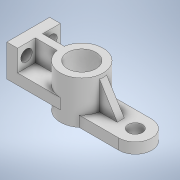
# Autodesk Inventor part: Exercise03
Saved by Autodesk Inventor 2021 (Build 250183000, 183)
## iProperties
Created: 2022-03-19
Part Number: Exercise03
Material: Generic
Document SubType Name: Modeling
Designer: User
Density: 1 g/cm^3
Appearance: Default
Author: User
Autodesk Inventor part; units mm, degrees
ref_plane "YZ Plane" through (0, 0, 0) normal (1, 0, 0) x (0, 1, 0)
ref_plane "XZ Plane" through (0, 0, 0) normal (0, 1, 0) x (-1, 0, 0)
ref_plane "XY Plane" through (0, 0, 0) normal (0, 0, 1) x (1, 0, 0)
sketch "Sketch1" plane through (0, 0, 0) normal (0, 1, 0) x (-1, 0, 0)
  circle A0 centre (0, 0) radius 30
  circle A1 centre (0, 0) radius 20
  dimension "d0" = 60
  dimension "d1" = 40
  constraints: 2 centre point, 2 coincident
  measures "d0" diameter of A0
  measures "d1" diameter of A1
extrude "Extrusion1" add sketch "Sketch1" along normal blind 60
sketch "Sketch2" plane through (0, 0, 0) normal (0, -1, 0) x (1, 0, 0)
  circle A0 centre (75, 0) radius 10
  arc A1 (75, -23) -> (75, 23) centre (75, 0) ccw
  circle A2 centre (0, 0) radius 30 projected
  line L0 (19.2614, 23) -> (75, 23)
  line L1 (19.2614, -23) -> (75, -23)
  dimension "d4" = 20
  dimension "d5" = 46
  dimension "d8" = 75
  constraints: 4 end point, 4 point on circle, 2 centre point, 2 parallel, 1 coincident, 1 horizontal, 1 horizontal alignment, 1 tangent
  measures "d4" diameter of A0
  measures "d5" diameter of A1
  measures "d8" distance of A1.centre A2.centre
extrude "Extrusion2" add sketch "Sketch2" against normal blind 15 contours L1 A2 L0 A1
sketch "Sketch3" plane through (0, 15, 0) normal (0, 1, 0) x (1, 0, 0)
  line L0 (-75, -30) -> (0, -30)
  line L1 (0, -30) -> (0, 30)
  line L2 (0, 30) -> (-75, 30)
  line L3 (-75, 30) -> (-75, -30)
  arc A0 (19.2614, 23) -> (19.2614, -23) centre (0, 0) ccw projected
  dimension "d11" = 60
  dimension "d12" = 75
  constraints: 8 end point, 2 parallel, 2 point on circle, 1 horizontal, 1 perpendicular
  measures "d11" distance of L2.end L0.start
  measures "d12" distance of L0.start L0.end
extrude "Extrusion3" add sketch "Sketch3" along normal blind 15 contours L3 L2 A0 L0
sketch "Sketch4" plane through (0, 30, 0) normal (0, 1, 0) x (1, 0, 0)
  line L0 (-75, 30) -> (-60, 30)
  line L1 (-60, 30) -> (-60, -30)
  line L2 (-60, -30) -> (-75, -30)
  line L3 (-75, -30) -> (-75, 30)
  line L4 (0, 30) -> (-75, 30) projected
  line L5 (-75, 30) -> (-75, -30) projected
  line L6 (-75, -30) -> (0, -30) projected
  line L7 (-60, 5) -> (-29.5804, 5)
  line L8 (-29.5804, 5) -> (-29.5804, -5)
  line L9 (-29.5804, -5) -> (-60, -5)
  line L10 (-60, -5) -> (-60, 5)
  circle A0 centre (0, 0) radius 30 projected
  dimension "d15" = 15
  dimension "d16" = 10
  constraints: 16 end point, 4 parallel, 3 collinear, 2 horizontal, 2 perpendicular, 2 point on circle, 1 point on line
  measures "d15" distance between parallel lines of L3 L1
  measures "d16" distance between parallel lines of L7 L9
extrude "Extrusion4" add sketch "Sketch4" along normal blind 30 contours L0 L1 L2 L3 | L7 A0 L9 L1 | L8 A0 picked at (-29.7047, 0.5579)
sketch "Sketch5" plane through (-75, 15, -30) normal (-1, 0, 0) x (0, 0, 1)
  circle A0 centre (12.5, 30) radius 8
  circle A1 centre (47.5, 30) radius 8
  line L0 (60, 0) -> (60, 45) projected
  line L1 (0, 45) -> (60, 45) projected
  point P0 (30, -15)
  dimension "d19" = 16
  dimension "d20" = 35
  dimension "d21" = 12.5
  dimension "d22" = 15
  constraints: 2 centre point, 1 equal radius, 1 horizontal alignment
  measures "d19" diameter of A0
  measures "d20" distance of A1.centre A0.centre
  measures "d21" distance from line of L0 A1.centre
  measures "d22" distance from line of L1 A0.centre
extrude "Extrusion5" cut sketch "Sketch5" against normal up to surface (15 mm away)
sketch "Sketch6" plane through (0, 0, 0) normal (0, 0, 1) x (1, 0, 0)
  line L0 (29.615, 55) -> (29.615, 15)
  line L1 (29.615, 15) -> (54.615, 15)
  line L2 (54.615, 15) -> (29.615, 55)
  line L3 (19.2614, 15) -> (75, 15) projected
  line L4 (29.998, 59.9996) -> (29.998, 15) construction
  point P0 (0, 0)
  dimension "d25" = 25
  dimension "d26" = 40
  dimension "d27" = 0.383
  constraints: 8 end point, 2 perpendicular, 1 point on line, 1 vertical
  measures "d25" distance of L0.end L1.end
  measures "d26" distance of L0.start L0.end
  measures "d27" distance between parallel lines of L4 L0
extrude "Extrusion6" add sketch "Sketch6" along normal mid plane 10
body "Solid1"
